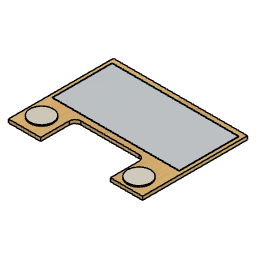
Aesthetic-design_Drive_Through_Design (Autodesk Fusion 360 design; units mm, degrees)
Autodesk Fusion 360 part; units mm, degrees
sketch "Sketch1" plane through (0, 0, 0) normal (0, 1, 0) x (1, 0, 0)
  line L0 (-25, 25) -> (-25, 482)
  line L1 (-25, 482) -> (-609, 482)
  line L2 (-609, 482) -> (-609, 25)
  line L3 (-609, 25) -> (-469, 25)
  line L4 (-444, 175) -> (-190, 175)
  line L5 (-469, 25) -> (-469, 150)
  arc A0 (-444, 175) -> (-469, 150) centre (-444, 150) ccw
  line L6 (-165, 25) -> (-25, 25)
  line L7 (-165, 150) -> (-165, 25)
  arc A1 (-165, 150) -> (-190, 175) centre (-190, 150) ccw
  point P0 (-469, 175)
  point P1 (-165, 175)
  dimension "d1" = 457
  dimension "d2" = 584
  dimension "d3" = 457
  dimension "d5" = 304
  dimension "d7" = 25
  dimension "d8" = 25
  constraint vertical L0
  constraint perpendicular L0 L1
  constraint perpendicular L1 L2
  constraint perpendicular L2 L3
  constraint perpendicular L4 L5
  constraint coincident P0 L4
  constraint coincident P0 L5
  constraint tangent L4 A0
  constraint tangent L5 A0
  constraint perpendicular L0 L6
  constraint perpendicular L6 L7
  constraint coincident P1 L4
  constraint coincident P1 L7
  constraint tangent L4 A1
  constraint tangent L7 A1
  measures "d1" distance of L0.start L0.end
  measures "d2" distance of L0.end L1.end
  measures "d3" distance of L1.end L2.end
  measures "d5" distance of P0 P1
  measures "d7" radius of A0
  measures "d8" radius of A1
extrude "Extrude1" add sketch "Sketch1" along normal blind 15 makes body 1
sketch "Sketch2" plane through (0, 15, 0) normal (0, 1, 0) x (-1, 0, 0)
  line L0 (165, -25) -> (25, -25)
  line L1 (25, -25) -> (25, -482)
  line L2 (25, -482) -> (609, -482)
  line L3 (609, -482) -> (609, -25)
  line L4 (609, -25) -> (469, -25)
  line L5 (469, -25) -> (469, -150)
  arc A0 (444, -175) -> (469, -150) centre (444, -150) ccw
  line L6 (444, -175) -> (190, -175)
  arc A1 (165, -150) -> (190, -175) centre (190, -150) ccw
  line L7 (165, -150) -> (165, -25)
  circle A2 centre (103.3226, -87.5) radius 50
  dimension "d11" = 100
  measures "d11" diameter of A2
extrude "Extrude2" add sketch "Sketch2" along normal blind 5 contours A2 bodies 1
sketch "Sketch3" plane through (0, 20, 0) normal (0, 1, 0) x (-1, 0, 0)
  circle A0 centre (103.3226, -87.5) radius 50
  circle A1 centre (540, -100) radius 50
  dimension "d14" = 100
  measures "d14" diameter of A1
extrude "Extrude3" add sketch "Sketch3" along normal blind 5 separate body contours A1 makes body 2
sketch "Sketch4" plane through (0, 15, 0) normal (0, 1, 0) x (-1, 0, 0)
  circle A0 centre (103.3226, -87.5) radius 50
  line L0 (165, -25) -> (25, -25)
  line L1 (25, -25) -> (25, -482)
  line L2 (25, -482) -> (609, -482)
  line L3 (609, -482) -> (609, -25)
  line L4 (609, -25) -> (469, -25)
  line L5 (469, -25) -> (469, -150)
  arc A1 (444, -175) -> (469, -150) centre (444, -150) ccw
  line L6 (444, -175) -> (190, -175)
  arc A2 (165, -150) -> (190, -175) centre (190, -150) ccw
  line L7 (165, -150) -> (165, -25)
  line L8 (592.6486, -459.5609) -> (40.3845, -459.5609)
  line L9 (40.3845, -459.5609) -> (40.3845, -199.9999)
  line L10 (40.3845, -199.9999) -> (592.6486, -199.9999)
  line L11 (592.6486, -199.9999) -> (592.6486, -459.5609)
  dimension "d17" = 259.561
  constraint horizontal L8
  constraint vertical L9
  constraint horizontal L10
  constraint vertical L11
  measures "d17" distance of L8.start L10.end
extrude "Extrude4" add sketch "Sketch4" along normal blind 2 contours L8 L9 L10 L11 bodies 1
